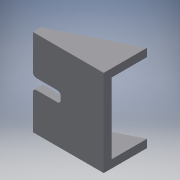
# Autodesk Inventor part: wire lead
Saved by Autodesk Inventor 2018 (Build 220112000, 112)
## iProperties
Created: 2018-06-15
Part Number: wire lead
Material: 一般
Document SubType Name: Modeling
Designer: KITformula
Density: 1 g/cm^3
Appearance: 既定
Author: KITformula
Autodesk Inventor part; units mm, degrees
ref_plane "YZ Plane" through (0, 0, 0) normal (1, 0, 0) x (0, 1, 0)
ref_plane "XZ Plane" through (0, 0, 0) normal (0, 1, 0) x (-1, 0, 0)
ref_plane "XY Plane" through (0, 0, 0) normal (0, 0, 1) x (1, 0, 0)
sketch "スケッチ1" plane through (0, 0, 0) normal (1, 0, 0) x (0, 1, 0)
  line L0 (-12.5, 12.5) -> (12.5, 12.5)
  line L1 (12.5, 12.5) -> (12.5, -12.5)
  line L2 (12.5, -12.5) -> (-12.5, -12.5)
  line L3 (-12.5, -12.5) -> (-12.5, 12.5)
  line L4 (-12.5, 12.5) -> (12.5, -12.5) construction
  line L5 (12.5, 12.5) -> (-12.5, -12.5) construction
  line L6 (10.2, 10.2) -> (-10.2, 10.2)
  line L7 (-10.2, 10.2) -> (-10.2, -10.2)
  line L8 (-10.2, -10.2) -> (10.2, -10.2)
  line L9 (10.2, -10.2) -> (10.2, 10.2)
  point P0 (0, 0)
  dimension "d0" = 25
  dimension "d1" = 25
  dimension "d2" = 2.3
  constraints: 20 end point, 4 parallel, 2 midpoint, 2 perpendicular, 1 horizontal, 3 other
  measures "d0" distance of L0.start L0.end
  measures "d1" distance of L2.end L0.start
  measures "d2" distance between parallel lines of L0 L6
extrude "押し出し1" add sketch "スケッチ1" along normal blind 25
sketch "スケッチ2" plane through (0, -12.5, 12.5) normal (0, 0, 1) x (1, 0, 0)
  line L0 (25, 25) -> (25, 0) projected
  line L1 (0, 12.5) -> (25, 12.5)
  line L2 (25, 12.5) -> (25, 25)
  line L3 (25, 25) -> (0, 25)
  line L4 (0, 25) -> (0, 12.5)
  constraints: 8 end point, 2 parallel, 1 horizontal, 1 perpendicular
extrude "押し出し2" cut sketch "スケッチ2" against normal through all
sketch "スケッチ3" plane through (0, -12.5, 12.5) normal (0, 0, 1) x (1, 0, 0)
  line L0 (0, 0) -> (0, 12.5) projected
  line L1 (0, 0) -> (25, 12.5)
  line L2 (25, 12.5) -> (0, 12.5) projected
  constraints: 2 end point, 1 coincident
extrude "押し出し3" cut sketch "スケッチ3" against normal through all
sketch "スケッチ4" plane through (25, -10.2, 10.2) normal (0, 1, 0) x (1, 0, 0)
  line L0 (-25, -2.3) -> (0, -2.3) projected
  line L1 (-25, 22.7) -> (0, 22.7) projected
  line L2 (-25, -2.3) -> (-20.4, -2.3)
  line L3 (-20.4, -2.3) -> (-20.4, 22.7)
  line L4 (-20.4, 22.7) -> (-25, 22.7)
  line L5 (-25, 22.7) -> (-25, -2.3)
  line L6 (-20.4, 20.4) -> (-20.4, 0) projected
  point P0 (-25, 10.2)
  constraints: 8 end point, 2 parallel, 1 collinear, 1 horizontal, 1 perpendicular, 1 point on line
extrude "押し出し4" cut sketch "スケッチ4" against normal blind 10
sketch "スケッチ5" plane through (25, -10.2, 10.2) normal (0, 1, 0) x (1, 0, 0)
  line L0 (-20.4, 8.7) -> (-12.9, 8.7)
  line L1 (-12.9, 8.7) -> (-12.9, 11.7)
  line L2 (-12.9, 11.7) -> (-20.4, 11.7)
  line L3 (-20.4, 11.7) -> (-20.4, 8.7)
  line L4 (-20.4, 20.4) -> (-20.4, 0) projected
  point P0 (-25, 10.2)
  point P1 (-20.4, 10.2)
  dimension "d11" = 3
  dimension "d12" = 7.5
  constraints: 8 end point, 2 midpoint, 2 parallel, 1 collinear, 1 horizontal, 1 perpendicular
  measures "d11" distance of L2.end L0.start
  measures "d12" distance of L1.end L2.end
extrude "押し出し5" cut sketch "スケッチ5" against normal blind 10
fillet "フィレット1" radius 1 4 edges at (4.6, -11.35, -1.5) (4.6, -11.35, 1.5) (12.1, -11.35, -1.5) (12.1, -11.35, 1.5)
equation "\"d1\" = d0"
